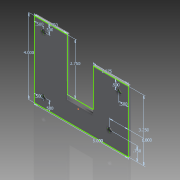
# Autodesk Inventor part: AS5-8-4-001
Saved by Autodesk Inventor 2011 SP1 (Build 150282100, 282)
## iProperties
Created: 2011-01-12
Part Number: AS5-8-4-001
Document SubType Name: Modeling
Designer: Christopher
Density: 1 g/cm^3
Author: Christopher
Autodesk Inventor part; units mm, degrees
ref_plane "YZ Plane" through (0, 0, 0) normal (1, 0, 0) x (0, 1, 0)
ref_plane "XZ Plane" through (0, 0, 0) normal (0, 1, 0) x (-1, 0, 0)
ref_plane "XY Plane" through (0, 0, 0) normal (0, 0, 1) x (1, 0, 0)
sketch "Sketch1" plane through (0, 0, 0) normal (0, 0, 1) x (1, 0, 0)
  line L0 (-59.7338, 79.3295) -> (-59.7338, -22.2705)
  line L1 (-59.7338, -22.2705) -> (67.2662, -22.2705)
  line L2 (67.2662, -22.2705) -> (67.2662, 60.2795)
  line L3 (67.2662, 60.2795) -> (19.6412, 60.2795)
  line L4 (19.6412, 60.2795) -> (19.6412, 9.4795)
  line L5 (19.6412, 9.4795) -> (-15.2838, 9.4795)
  line L6 (-15.2838, 9.4795) -> (-15.2838, 79.3295)
  line L7 (-15.2838, 79.3295) -> (-59.7338, 79.3295)
  point P0 (0, 0)
  point P1 (-47.0338, 66.6295)
  point P2 (54.5662, 47.5795)
  point P3 (41.8662, -3.2205)
  point P4 (-47.0338, -9.5705)
  dimension "d0" = 101.6
  dimension "d1" = 127
  dimension "d2" = 44.45
  dimension "d3" = 47.625
  dimension "d4" = 82.55
  dimension "d5" = 69.85
  dimension "d6" = 12.7
  dimension "d7" = 12.7
  dimension "d8" = 12.7
  dimension "d9" = 12.7
  dimension "d10" = 19.05
  dimension "d11" = 25.4
  dimension "d21" = 12.7
  dimension "d22" = 12.7
  constraints: 16 end point, 6 parallel, 1 perpendicular, 1 vertical
  measures "d0" distance of L0.start L0.end
  measures "d1" distance of L0.end L1.end
  measures "d2" distance of L6.end L0.start
  measures "d3" distance of L2.end L3.end
  measures "d4" distance of L1.end L2.end
  measures "d5" distance between parallel lines of L7 L5
  measures "d6" distance from line of L7 point (-47.034, 66.63)
  measures "d7" distance from line of L0 point (-47.034, 66.63)
  measures "d8" distance from line of L2 point (54.566, 47.58)
  measures "d9" distance from line of L3 point (54.566, 47.58)
  measures "d10" distance from line of L1 point (41.866, -3.22)
  measures "d11" distance from line of L2 point (41.866, -3.22)
  measures "d21" distance from line of L0 point (-47.034, -9.57)
  measures "d22" distance from line of L1 point (-47.034, -9.57)
extrude "Extrusion1" add sketch "Sketch1" against normal blind 3.175
hole "Hole1" at (-47.0338, 66.6295, 0) at (54.5662, 47.5795, 0) at (41.8662, -3.2205, 0) direction (0, 0, -1) diameter 6.35 depth 25.4 tip angle 118
hole "Hole2" at (-47.0338, -9.5705, 0) direction (0, 0, -1) diameter 6.35 end through all
body "Solid1"
